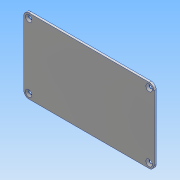
# Autodesk Inventor part: AK-C-C39-Bottom
Saved by Autodesk Inventor 2016 (Build 200138000, 138)
## iProperties
Created: 2016-04-01
Part Number: AK-C-C39-Bottom
Material: Aluminum 6061
Document SubType Name: Modeling
Designer: admin
Density: 2.7 g/cm^3
Appearance: Aluminum - Flat
Author: admin
Autodesk Inventor part; units mm, degrees
ref_plane "YZ Plane" through (0, 0, 0) normal (1, 0, 0) x (0, 1, 0)
ref_plane "XZ Plane" through (0, 0, 0) normal (0, 1, 0) x (-1, 0, 0)
ref_plane "XY Plane" through (0, 0, 0) normal (0, 0, 1) x (1, 0, 0)
derived "AK-C-C39-Main-Board.ipt"
sketch "Sketch1" plane through (0, 0, 0) normal (0, 1, 0) x (-1, 0, 0)
  line L0 (-55, -17.425) -> (-56.5, -17.425)
  line L1 (-56.5, -17.425) -> (-56.5, -16.775)
  line L2 (-58.5, -16.775) -> (-58.5, -17.425)
  line L3 (-58.5, -17.425) -> (-60, -17.425)
  line L4 (-60, -29.925) -> (-60, -17.425)
  line L5 (-60, -16.775) -> (-60, 29.925)
  line L6 (55, -17.425) -> (56.5, -17.425)
  line L7 (58.5, -17.425) -> (60, -17.425)
  line L8 (60, -29.925) -> (60, -17.425)
  line L9 (60, -16.775) -> (60, 29.925)
  arc A0 (-52.7, -29.3928) -> (-53.5536, -29.0392) centre (-53.2, -29.3928) ccw
  arc A1 (-54.6142, -27.9786) -> (-54.9678, -27.125) centre (-54.9678, -27.625) ccw
  line L10 (-54.0511, -29.5368) -> (-53.5536, -29.0392)
  line L11 (-55.1118, -28.4761) -> (-54.6142, -27.9786)
  arc A2 (54.6142, 27.9786) -> (54.9678, 27.125) centre (54.9678, 27.625) ccw
  line L12 (55.5, 29.925) -> (49.0175, 23.4425) construction
  arc A3 (52.7, 29.3928) -> (53.5536, 29.0392) centre (53.2, 29.3928) ccw
  line L13 (55, -16.775) -> (56.5, -16.775)
  line L14 (58.5, -16.775) -> (60, -16.775)
  line L15 (57.8, -3.3607) -> (55, -7.6074)
  line L16 (55, -7.6074) -> (55, -16.775)
  arc A4 (56.5, -18.525) -> (58.5, -18.525) centre (57.5, -19.275) ccw
  line L17 (58.5, -18.525) -> (58.5, -16.775)
  line L18 (56.5, -18.525) -> (56.5, -16.775)
  line L19 (-55.1118, 28.4761) -> (-54.6142, 27.9786)
  line L20 (-54.0059, 29.7916) -> (-53.5536, 29.3392)
  arc A5 (-53.5536, 29.3392) -> (-52.7, 29.6928) centre (-53.2, 29.6928) ccw
  arc A6 (-54.9678, 27.125) -> (-54.6142, 27.9786) centre (-54.9678, 27.625) ccw
  line L21 (-57.8, -3.3607) -> (-55, -7.6074)
  line L22 (-55, -7.6074) -> (-55, -16.775)
  arc A7 (-56.5, -15.025) -> (-58.5, -15.025) centre (-57.5, -14.275) ccw
  line L23 (-58.5, -15.025) -> (-58.5, -16.775)
  line L24 (-56.5, -15.025) -> (-56.5, -16.775)
  line L25 (-55, -16.775) -> (-56.5, -16.775)
  line L26 (-58.5, -16.775) -> (-60, -16.775)
  line L27 (57.5, -16.4962) -> (57.5, -11.7384) construction
  line L28 (-52.7, -31.925) -> (-52.7, -29.3928)
  line L29 (-54.9678, -27.125) -> (-57.5, -27.125)
  line L30 (-57.5, -27.125) -> (-57.5, -25.125)
  line L31 (-57.5, -25.125) -> (-55, -25.125)
  line L32 (-55, -25.125) -> (-55, -17.425)
  line L33 (48.7, -31.925) -> (46.7, -31.925)
  line L34 (46.7, -31.925) -> (46.7, -29.925)
  line L35 (46.7, -29.925) -> (44.7, -29.925)
  line L36 (44.7, -29.925) -> (44.7, -32.225)
  line L37 (-44.7, -32.225) -> (-44.7, -29.925)
  line L38 (-44.7, -29.925) -> (-46.7, -29.925)
  line L39 (-46.7, -29.925) -> (-46.7, -31.925)
  line L40 (-46.7, -31.925) -> (-48.7, -31.925)
  line L41 (-48.7, -31.925) -> (-48.7, -29.925)
  line L42 (-48.7, -29.925) -> (-50.7, -29.925)
  line L43 (-50.7, -29.925) -> (-50.7, -31.925)
  line L44 (-50.7, -31.925) -> (-52.7, -31.925)
  line L45 (55, -17.425) -> (55, -25.125)
  line L46 (55, -25.125) -> (57.5, -25.125)
  line L47 (57.5, -25.125) -> (57.5, -27.125)
  line L48 (57.5, -27.125) -> (54.9678, -27.125)
  line L49 (52.7, -29.3928) -> (52.7, -31.925)
  line L50 (52.7, -31.925) -> (50.7, -31.925)
  line L51 (50.7, -31.925) -> (50.7, -29.925)
  line L52 (50.7, -29.925) -> (48.7, -29.925)
  line L53 (48.7, -29.925) -> (48.7, -31.925)
  line L54 (5, -32.225) -> (5, -29.925)
  line L55 (5, -29.925) -> (3, -29.925)
  line L56 (3, -29.925) -> (3, -31.925)
  line L57 (3, -31.925) -> (1, -31.925)
  line L58 (1, -31.925) -> (1, -29.925)
  line L59 (1, -29.925) -> (-1, -29.925)
  line L60 (-1, -29.925) -> (-1, -31.925)
  line L61 (-1, -31.925) -> (-3, -31.925)
  line L62 (-3, -31.925) -> (-3, -29.925)
  line L63 (-3, -29.925) -> (-5, -29.925)
  line L64 (-5, -29.925) -> (-5, -32.225)
  line L65 (-5, -32.225) -> (-44.7, -32.225)
  line L66 (44.7, -32.225) -> (5, -32.225)
  line L67 (-57.5, -20.9142) -> (-57.5, -16.6435) construction
  arc A8 (60, 29.925) -> (55.5, 34.425) centre (55.5, 29.925) ccw
  arc A9 (-55.5, 34.425) -> (-60, 29.925) centre (-55.5, 29.925) ccw
  arc A10 (-60, -29.925) -> (-55.5, -34.425) centre (-55.5, -29.925) ccw
  line L68 (57.5, 27.125) -> (57.5, 25.125)
  line L69 (57.5, 25.125) -> (55.5, 25.125)
  line L70 (55.5, 25.125) -> (55.5, 23.125)
  line L71 (55.5, 23.125) -> (57.5, 23.125)
  line L72 (57.5, 23.125) -> (57.5, 21.125)
  line L73 (57.5, 21.125) -> (55.5, 21.125)
  line L74 (55.5, 21.125) -> (55.5, 19.125)
  line L75 (55.5, 19.125) -> (57.8, 19.125)
  line L76 (57.8, 19.125) -> (57.8, -3.3607)
  line L77 (3, 31.925) -> (1, 31.925)
  line L78 (1, 31.925) -> (1, 29.925)
  line L79 (1, 29.925) -> (-1, 29.925)
  line L80 (-1, 29.925) -> (-1, 31.925)
  line L81 (-1, 31.925) -> (-3, 31.925)
  line L82 (-3, 31.925) -> (-3, 29.925)
  line L83 (-3, 29.925) -> (-5, 29.925)
  line L84 (-5, 29.925) -> (-5, 32.225)
  line L85 (-5, 32.225) -> (-44.7, 32.225)
  line L86 (-44.7, 32.225) -> (-44.7, 29.925)
  line L87 (-44.7, 29.925) -> (-46.7, 29.925)
  line L88 (-46.7, 29.925) -> (-46.7, 32.225)
  line L89 (-46.7, 32.225) -> (-48.7, 32.225)
  line L90 (-48.7, 32.225) -> (-48.7, 29.925)
  line L91 (-48.7, 29.925) -> (-50.7, 29.925)
  line L92 (-50.7, 29.925) -> (-50.7, 32.225)
  line L93 (-50.7, 32.225) -> (-52.7, 32.225)
  line L94 (-52.7, 32.225) -> (-52.7, 29.6928)
  line L95 (-54.9678, 27.125) -> (-57.5, 27.125)
  line L96 (55.1118, 28.4761) -> (54.6142, 27.9786)
  line L97 (54.0511, 29.5368) -> (53.5536, 29.0392)
  line L98 (57.5, 27.125) -> (54.9678, 27.125)
  line L99 (52.7, 29.3928) -> (52.7, 31.925)
  line L100 (52.7, 31.925) -> (50.7, 31.925)
  line L101 (50.7, 31.925) -> (50.7, 29.925)
  line L102 (50.7, 29.925) -> (48.7, 29.925)
  line L103 (48.7, 29.925) -> (48.7, 31.925)
  line L104 (48.7, 31.925) -> (46.7, 31.925)
  line L105 (46.7, 31.925) -> (46.7, 29.925)
  line L106 (46.7, 29.925) -> (44.7, 29.925)
  line L107 (44.7, 29.925) -> (44.7, 32.225)
  line L108 (44.7, 32.225) -> (5, 32.225)
  line L109 (5, 32.225) -> (5, 29.925)
  line L110 (5, 29.925) -> (3, 29.925)
  line L111 (3, 29.925) -> (3, 31.925)
  line L112 (-57.5, 27.125) -> (-57.5, 25.125)
  line L113 (-57.5, 25.125) -> (-55.5, 25.125)
  line L114 (-55.5, 25.125) -> (-55.5, 23.125)
  line L115 (-55.5, 23.125) -> (-57.5, 23.125)
  line L116 (-57.5, 23.125) -> (-57.5, 21.125)
  line L117 (-57.5, 21.125) -> (-55.5, 21.125)
  line L118 (-55.5, 21.125) -> (-55.5, 19.125)
  line L119 (-55.5, 19.125) -> (-57.8, 19.125)
  line L120 (-57.8, 19.125) -> (-57.8, -3.3607)
  line L121 (55.5, -34.425) -> (-55.5, -34.425)
  line L122 (33.1179, 0) -> (-42.957, 0) construction
  line L123 (0, -20.0068) -> (0, 12.0803) construction
  line L124 (-77.7331, -29.925) -> (-117.8042, -29.925) construction
  line L125 (-91.6184, 29.925) -> (-122.9166, 29.925) construction
  line L126 (55.5, -18.8016) -> (55.5, 12.0803) construction
  line L127 (-55.5, -18.8016) -> (-55.5, 16.5996) construction
  arc A11 (55.5, -34.425) -> (60, -29.925) centre (55.5, -29.925) ccw
  arc A12 (54.9678, -27.125) -> (54.6142, -27.9786) centre (54.9678, -27.625) ccw
  arc A13 (53.5536, -29.0392) -> (52.7, -29.3928) centre (53.2, -29.3928) ccw
  line L128 (54.6142, -27.9786) -> (55.1118, -28.4761)
  line L129 (53.5536, -29.0392) -> (54.0511, -29.5368)
  arc A14 (55.1118, 28.4761) -> (54.0511, 29.5368) centre (55.5, 29.925) ccw
  arc A15 (-54.0059, 29.7916) -> (-55.1118, 28.4761) centre (-55.5, 29.925) ccw
  arc A16 (54.0511, -29.5368) -> (55.1118, -28.4761) centre (55.5, -29.925) ccw
  arc A17 (-55.1118, -28.4761) -> (-54.0511, -29.5368) centre (-55.5, -29.925) ccw
  line L130 (55.5, 34.425) -> (-55.5, 34.425)
  point P0 (0, 0)
sketch "Sketch2" plane through (0, 0, 0) normal (0, 1, 0) x (-1, 0, 0)
  line L0 (60, -29.925) -> (60, -17.425) projected
  arc A0 (55.5, -34.425) -> (60, -29.925) centre (55.5, -29.925) ccw projected
  line L1 (55.5, -34.425) -> (-55.5, -34.425) projected
  arc A1 (-60, -29.925) -> (-55.5, -34.425) centre (-55.5, -29.925) ccw projected
  line L2 (-60, -29.925) -> (-60, -17.425) projected
  line L3 (-60, -16.775) -> (-60, 29.925) projected
  arc A2 (-55.5, 34.425) -> (-60, 29.925) centre (-55.5, 29.925) ccw projected
  line L4 (55.5, 34.425) -> (-55.5, 34.425) projected
  arc A3 (60, 29.925) -> (55.5, 34.425) centre (55.5, 29.925) ccw projected
  line L5 (60, -16.775) -> (60, 29.925) projected
  line L6 (60, -17.425) -> (60, -16.775)
  line L7 (-60, -17.425) -> (-60, -16.775)
  point P0 (0, 0)
  constraints: 4 end point, 1 parallel, 1 vertical
extrude "Extrusion1" add sketch "Sketch2" along normal blind 2
hole "Hole1" at (-55.5, 0, 29.925) at (55.5, 0, 29.925) at (-55.5, 0, -29.925) at (55.5, 0, -29.925) direction (0, 1, 0) diameter 3 end through all countersink diameter 6 countersink angle 90
body "Solid1"
